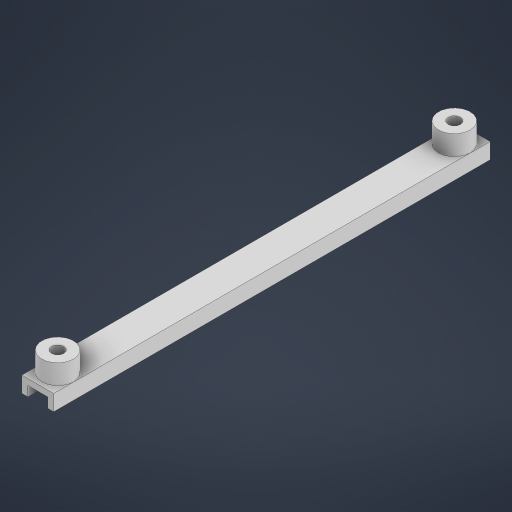
# Autodesk Inventor part: arm_xbrace_jig
Saved by Autodesk Inventor 2024 (Build 280153000, 153)
## iProperties
Created: 2024-01-19
Part Number: arm_xbrace_jig
Material: Generic
Document SubType Name: Modeling
Designer: avere
Density: 1 g/cm^3
Appearance: Default
Author: avere
Autodesk Inventor part; units mm, degrees
ref_plane "YZ Plane" through (0, 0, 0) normal (1, 0, 0) x (0, 1, 0)
ref_plane "XZ Plane" through (0, 0, 0) normal (0, 1, 0) x (-1, 0, 0)
ref_plane "XY Plane" through (0, 0, 0) normal (0, 0, 1) x (1, 0, 0)
sketch "Sketch1" plane through (0, 0, 0) normal (0, 0, 1) x (1, 0, 0)
  line L0 (3.175, 0) -> (3.175, 3.175)
  line L1 (3.175, 3.175) -> (-3.175, 3.175)
  line L2 (-3.175, 3.175) -> (-3.175, 0)
  line L3 (5.08, 0) -> (5.08, 5.08)
  line L4 (5.08, 5.08) -> (-5.08, 5.08)
  line L5 (-5.08, 5.08) -> (-5.08, 0)
  line L6 (-5.08, 0) -> (-3.175, 0)
  line L7 (3.175, 0) -> (5.08, 0)
  point P0 (0, 0)
  dimension "d0" = 10.16
  dimension "d1" = 5.08
  constraints: 16 end point, 4 parallel, 2 horizontal, 2 perpendicular
  measures "d0" distance of L4.end L3.end
  measures "d1" distance of L3.end L3.start
extrude "Extrusion1" add sketch "Sketch1" along normal blind 139.7
sketch "Sketch2" plane through (-5.08, 5.08, 0) normal (0, 1, 0) x (1, 0, 0)
  circle A0 centre (5.08, -6.35) radius 1.9844
  circle A1 centre (5.08, -133.35) radius 1.9844
  point P0 (5.08, 0)
  dimension "d4" = 3.9688
  dimension "d5" = 3.9688
  constraints: 2 centre point
  measures "d4" diameter of A0
  measures "d5" diameter of A1
extrude "Extrusion2" cut sketch "Sketch2" against normal blind 139.7
sketch "Sketch3" plane through (-5.08, 5.08, 0) normal (0, 1, 0) x (1, 0, 0)
  circle A0 centre (5.08, -6.35) radius 1.9844 projected
  circle A1 centre (5.08, -133.35) radius 1.9844 projected
  circle A2 centre (5.08, -133.35) radius 5.08
  line L0 (0, 0) -> (0, -139.7) projected
  circle A3 centre (5.08, -6.35) radius 5.08
  point P0 (5.08, 0)
  constraints: 2 centre point, 2 coincident, 2 tangent
extrude "Extrusion3" add sketch "Sketch3" along normal blind 6.35
body "Solid1"
